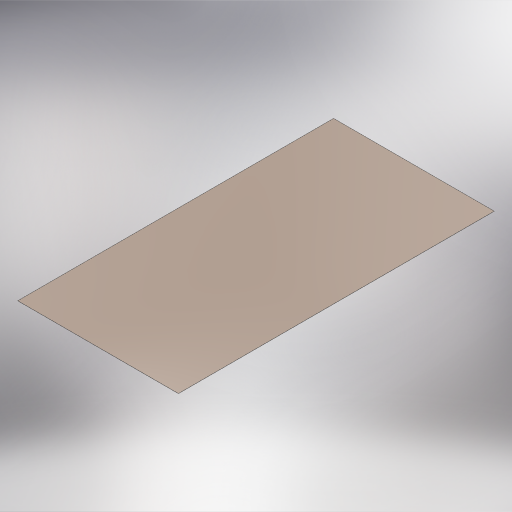
# Autodesk Inventor part: Kapton Cover
Saved by Autodesk Inventor 2024 (Build 280153000, 153)
## iProperties
Created: 2024-03-28
Part Number: Kapton Cover
Material: Generic
Document SubType Name: Modeling
Designer: cfang
Density: 1 g/cm^3
Appearance: Default
Author: cfang
Autodesk Inventor part; units mm, degrees
ref_plane "YZ Plane" through (0, 0, 0) normal (1, 0, 0) x (0, 1, 0)
ref_plane "XZ Plane" through (0, 0, 0) normal (0, 1, 0) x (-1, 0, 0)
ref_plane "XY Plane" through (0, 0, 0) normal (0, 0, 1) x (1, 0, 0)
sketch "Sketch1" plane through (0, 0, 0) normal (0, 1, 0) x (-1, 0, 0)
  line L0 (-14.5, -28.5) -> (14.5, -28.5)
  line L1 (14.5, -28.5) -> (14.5, 28.5)
  line L2 (14.5, 28.5) -> (-14.5, 28.5)
  line L3 (-14.5, 28.5) -> (-14.5, -28.5)
  line L4 (-14.5, -28.5) -> (14.5, 28.5) construction
  line L5 (14.5, -28.5) -> (-14.5, 28.5) construction
  point P0 (0, 0)
  dimension "d0" = 29
  dimension "d1" = 57
  constraints: 12 end point, 2 midpoint, 2 parallel, 1 horizontal, 1 perpendicular
  measures "d0" distance of L1.end L2.end
  measures "d1" distance of L0.end L1.end
extrude "Extrusion1" add sketch "Sketch1" along normal blind 0.025
body "Solid1"
